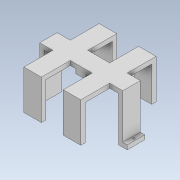
# Autodesk Inventor part: battery_fix
Saved by Autodesk Inventor 2020 (Build 240168000, 168)
## iProperties
Created: 2021-02-09
Part Number: battery_fix
Material: Generic
Document SubType Name: Modeling
Designer: DELL
Density: 1 g/cm^3
Appearance: Default
Author: DELL
Autodesk Inventor part; units mm, degrees
ref_plane "YZ Plane" through (0, 0, 0) normal (1, 0, 0) x (0, 1, 0)
ref_plane "XZ Plane" through (0, 0, 0) normal (0, 1, 0) x (-1, 0, 0)
ref_plane "XY Plane" through (0, 0, 0) normal (0, 0, 1) x (1, 0, 0)
sketch "Sketch1" plane through (0, 0, 0) normal (0, 0, 1) x (1, 0, 0)
  line L0 (-52.5, 5) -> (-47.5, 5)
  line L1 (-47.5, 5) -> (-47.5, 56)
  line L2 (-47.5, 56) -> (47.5, 56)
  line L3 (47.5, 56) -> (47.5, 5)
  line L4 (47.5, 5) -> (52.5, 5)
  line L5 (-42.5, 0) -> (-42.5, 51)
  line L6 (-42.5, 51) -> (42.5, 51)
  line L7 (42.5, 51) -> (42.5, 0)
  line L8 (0, 0) -> (0, -25.7238) construction
  line L9 (52.5, 0) -> (52.5, 5)
  line L10 (-52.5, 0) -> (-52.5, 5)
  line L11 (-52.5, 0) -> (-42.5, 0)
  line L12 (42.5, 0) -> (52.5, 0)
  line L13 (-32.5, 56) -> (-12.5, 56)
  line L14 (-12.5, 56) -> (-12.5, 51)
  line L15 (-12.5, 51) -> (-32.5, 51)
  line L16 (-32.5, 51) -> (-32.5, 56)
  line L17 (12.5, 56) -> (32.5, 56)
  line L18 (32.5, 56) -> (32.5, 51)
  line L19 (32.5, 51) -> (12.5, 51)
  line L20 (12.5, 51) -> (12.5, 56)
  line L21 (-32.5, 56) -> (-12.5, 56)
  line L22 (-12.5, 56) -> (-12.5, 11)
  line L23 (-12.5, 11) -> (-32.5, 11)
  line L24 (-32.5, 11) -> (-32.5, 56)
  line L25 (12.5, 56) -> (32.5, 56)
  line L26 (32.5, 56) -> (32.5, 11)
  line L27 (32.5, 11) -> (12.5, 11)
  line L28 (12.5, 11) -> (12.5, 56)
  point P0 (32.5, 56)
  point P1 (-32.5, 51)
  point P2 (-12.5, 56)
  point P3 (32.5, 56)
  point P4 (-32.5, 56)
  dimension "d1" = 5
  dimension "d2" = 5
  dimension "d3" = 5
  dimension "d5" = 85
  dimension "d6" = 51
  dimension "d8" = 5
  dimension "d18" = 105
  dimension "d19" = 20
  dimension "d20" = 25
  dimension "d21" = 45
  constraints: 58 end point, 10 equal length, 8 perpendicular, 8 point on line, 7 horizontal, 3 collinear, 1 vertical, 4 other
  measures "d1" distance between parallel lines of L1 L5
  measures "d2" distance between parallel lines of L2 L6
  measures "d3" distance between parallel lines of L3 L7
  measures "d5" distance between parallel lines of L7 L5
  measures "d6" distance between parallel lines of L6 L11
  measures "d8" distance between parallel lines of L11 L0
  measures "d18" distance between parallel lines of L9 L10
  measures "d19" distance between parallel lines of L14 L16
  measures "d20" distance between parallel lines of L20 L14
  measures "d21" distance between parallel lines of L21 L23
extrude "Extrusion1" add sketch "Sketch1" along normal mid plane 20 contours L0 L1 L2 L16 L6 L5 L11 L10 | L2 L14 L6 L16 | L2 L20 L6 L14 | L2 L18 L6 L20 | L2 L3 L4 L9 L12 L7 L6 L18
sketch "Sketch2" plane through (-52.5, 0, 10) normal (0, -1, 0) x (1, 0, 0)
  circle A0 centre (2.5, -10) radius 1.25
  circle A1 centre (102.5, -10) radius 1.25
  line L0 (52.5, -10) -> (52.5, 0) construction
  line L1 (10, 0) -> (95, 0) construction
  circle A2 centre (2.5, -10) radius 2.25
  circle A3 centre (102.5, -10) radius 2.25
  dimension "d11" = 2.5
  dimension "d12" = 100
  dimension "d15" = 4.5
  constraints: 4 centre point, 2 coincident, 2 end point, 2 equal radius, 2 horizontal alignment, 1 midpoint, 1 symmetric about line
  measures "d11" diameter of A0
  measures "d12" distance of A1.centre A0.centre
  measures "d15" diameter of A3
extrude "Extrusion2" cut sketch "Sketch2" against normal through all contours A0 | A1
extrude "Extrusion4" add sketch "Sketch1" along normal blind 28 from surface at 10 contours L2 L14 L6 L16 | L2 L18 L6 L20
extrude "Extrusion5" add sketch "Sketch1" along normal blind 5 from surface at 38 contours L2 L14 L6 L16 | L6 L22 L23 L24 | L2 L18 L6 L20 | L6 L26 L27 L28
mirror "Mirror1" about plane through (0, 0, 0) normal (0, 0, 1) of "Extrusion5", "Extrusion4"
sketch "Sketch3" plane through (42.5, 51, -10) normal (0, -1, 0) x (1, 0, 0)
  line L0 (-55, 20) -> (-30, 20) projected
  line L1 (-36.5, 0) -> (-48.5, 0)
  line L2 (-48.5, 0) -> (-48.5, 20)
  line L3 (-48.5, 20) -> (-36.5, 20)
  line L4 (-36.5, 20) -> (-36.5, 0)
  line L5 (-36.5, 0) -> (-48.5, 20) construction
  line L6 (-48.5, 0) -> (-36.5, 20) construction
  point P0 (-42.5, 10)
  dimension "d26" = 12
  constraints: 12 end point, 2 midpoint, 2 parallel, 1 horizontal, 1 perpendicular, 1 point on line
  measures "d26" distance between parallel lines of L4 L2
extrude "Extrusion6" add sketch "Sketch3" along normal blind 5
equation "\"d1\" = d8"
equation "\"d2\" = d8"
equation "\"d3\" = d8"
body "Solid1"
